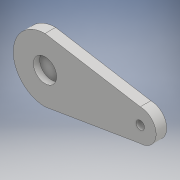
# Autodesk Inventor part: Part2
Saved by Autodesk Inventor 2018 (Build 220112000, 112)
## iProperties
Created: 2017-06-05
Part Number: Part2
Material: Generic
Document SubType Name: Modeling
Designer: Zadeka
Density: 1 g/cm^3
Appearance: Default
Author: Zadeka
Autodesk Inventor part; units mm, degrees
note: some values were not read from the file. Chosen so that the rebuilt part matches the saved one: sketch regions of "Extrusion1".
ref_plane "YZ Plane" through (0, 0, 0) normal (1, 0, 0) x (0, 1, 0)
ref_plane "XZ Plane" through (0, 0, 0) normal (0, 1, 0) x (-1, 0, 0)
ref_plane "XY Plane" through (0, 0, 0) normal (0, 0, 1) x (1, 0, 0)
sketch "Sketch1" plane through (0, 0, 0) normal (0, 1, 0) x (-1, 0, 0)
  circle A0 centre (0, 0) radius 22
  circle A1 centre (0, -22) radius 1.55
  circle A2 centre (0, -22) radius 3
  circle A3 centre (22, 0) radius 3
  circle A4 centre (22, 0) radius 1.55
  circle A5 centre (0, 22) radius 3
  circle A6 centre (0, 22) radius 1.55
  circle A7 centre (-22, 0) radius 3
  circle A8 centre (-22, 0) radius 1.55
  circle A9 centre (0, 0) radius 30
  circle A10 centre (-90, 0) radius 4
  circle A11 centre (-90, 0) radius 15
  line L0 (0, -30) -> (-90, -15)
  line L1 (0, 30) -> (-90, 15)
  circle A12 centre (0, 0) radius 5
  circle A13 centre (0, 0) radius 11
  dimension "d2" = 44
  dimension "d3" = 3.1
  dimension "d4" = 6
  dimension "d5" = 360
  dimension "d6" = 60
  dimension "d8" = 8
  dimension "d9" = 30
  dimension "d10" = 10
  dimension "d11" = 22
  constraints: 14 centre point, 9 coincident, 4 end point, 4 point on circle, 17 other
  measures "d2" diameter of A0
  measures "d3" diameter of A1
  measures "d4" diameter of A2
  measures "d6" diameter of A9
  measures "d8" diameter of A10
  measures "d9" diameter of A11
  measures "d10" diameter of A12
  measures "d11" diameter of A13
extrude "Extrusion1" add sketch "Sketch1" along normal blind 10 contours A0 A4 | A0 A4 | A4 A0 A3 | A0 A3 A4 | A3 A0 A2 A7 A5 | A5 A0 A6 | A0 A6 A5 | A2 A0 A1 | A0 A1 A2 | A6 A0 | A0 A6 | A1 A0 | A0 A1 | A7 A0 A8 | A0 A8 A7 | A8 A0 | A0 A8 | A9 L0 L1 | A9 L0 A11 L1 | A11
sketch "Sketch2" plane through (0, 10, 0) normal (0, 1, 0) x (1, 0, 0)
  circle A0 centre (0, 0) radius 11
  dimension "d14" = 22
  constraints: 1 centre point, 1 coincident
  measures "d14" diameter of A0
extrude "Extrusion2" add sketch "Sketch2" against normal blind 4
body "Solid1"
